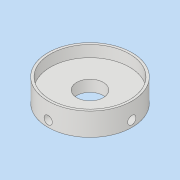
# Autodesk Inventor part: BallastThrustWasherSpacer
Saved by Autodesk Inventor 2017.3 (Build 213256000, 256)
## iProperties
Created: 2019-01-15
Part Number: BallastThrustWasherSpacer
Material: ABS Plastic
Document SubType Name: Modeling
Designer: Derek Wider
Density: 1.06 g/cm^3
Appearance: Smooth - White
Author: Derek Wider
Autodesk Inventor part; units mm, degrees
ref_plane "XZ Plane" through (0, 0, 0) normal (0, 1, 0) x (-1, 0, 0)
ref_plane "XY Plane" through (0, 0, 0) normal (0, 0, 1) x (1, 0, 0)
sketch "Sketch1" plane through (0, 0, 0) normal (0, 1, 0) x (-1, 0, 0)
  circle A0 centre (0, 0) radius 16.8275
  dimension "d0" = 33.655
  constraints: 1 centre point, 1 coincident
  measures "d0" diameter of A0
extrude "Extrusion1" add sketch "Sketch1" along normal blind 4.572
sketch "Sketch2" plane through (0, 4.572, 0) normal (0, 1, 0) x (1, 0, 0)
  circle A0 centre (0, 0) radius 15.875
  circle A1 centre (0, 0) radius 16.8275 projected
  dimension "d3" = 31.75
  constraints: 1 centre point, 1 coincident
  measures "d3" diameter of A0
extrude "Extrusion2" add sketch "Sketch2" along normal blind 4.572
ref_plane "Work Plane1" through (-16.8275, 0, 0) normal (1, 0, 0) x (0, 1, 0)
sketch "Sketch3" plane through (-16.8275, 0, 0) normal (1, 0, 0) x (0, 1, 0)
  circle A0 centre (2.54, 0) radius 1.651
  line L0 (0, 16.8275) -> (0, -16.8275) projected
  point P0 (0, 0)
  dimension "d6" = 3.302
  dimension "d7" = 2.54
  constraints: 1 centre point
  measures "d6" diameter of A0
  measures "d7" distance from line of L0 A0.centre
extrude "Extrusion3" cut sketch "Sketch3" along normal blind 2.413
pattern_circular "Circular Pattern1" count 4 over 360 about axis through (0, 0, 0) along (0, 1, 0) of "Extrusion3"
sketch "Sketch4" plane through (0, 4.572, 0) normal (0, 1, 0) x (1, 0, 0)
  circle A0 centre (0, 0) radius 5.334
  dimension "d13" = 10.668
  constraints: 1 centre point, 1 coincident
  measures "d13" diameter of A0
extrude "Extrusion4" cut sketch "Sketch4" against normal blind 25.4
body "Solid1"
